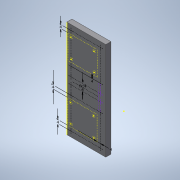
# Autodesk Inventor part: Z connection plate
Saved by Autodesk Inventor 2020 (Build 240168000, 168)
## iProperties
Created: 2019-05-25
Part Number: Z connection plate
Material: Generic
Document SubType Name: Modeling
Designer: LillaHunden
Density: 1 g/cm^3
Appearance: Default
Author: LillaHunden
Autodesk Inventor part; units mm, degrees
ref_plane "YZ Plane" through (0, 0, 0) normal (1, 0, 0) x (0, 1, 0)
ref_plane "XZ Plane" through (0, 0, 0) normal (0, 1, 0) x (-1, 0, 0)
ref_plane "XY Plane" through (0, 0, 0) normal (0, 0, 1) x (1, 0, 0)
sketch "Sketch1" plane through (0, 0, 0) normal (0, 0, 1) x (1, 0, 0)
  line L0 (-36.5524, -46.7459) -> (-66.2609, -46.7459) construction
  line L1 (-66.2609, -46.7459) -> (-66.2609, -56.6459) construction
  line L2 (-66.2609, -56.6459) -> (-1.9697, -56.6459) construction
  arc A0 (-1.9697, -56.6459) -> (0.0303, -54.6459) centre (-1.9697, -54.6459) ccw construction
  line L3 (0.0303, -54.6459) -> (0.0303, -27.2432) construction
  arc A1 (2.0303, -25.2432) -> (0.0303, -27.2432) centre (2.0303, -27.2432) ccw construction
  line L4 (2.0303, -25.2432) -> (9.9038, -25.2432) construction
  arc A2 (9.9038, -25.2432) -> (11.9038, -23.2432) centre (9.9038, -23.2432) ccw construction
  line L5 (11.9038, -23.2432) -> (11.9038, -14.7192) construction
  arc A3 (11.9038, -14.7192) -> (9.9038, -12.7192) centre (9.9038, -14.7192) ccw construction
  line L6 (9.9038, -12.7192) -> (2.0303, -12.7192) construction
  arc A4 (0.0303, -10.7192) -> (2.0303, -12.7192) centre (2.0303, -10.7192) ccw construction
  line L7 (0.0303, -10.7192) -> (0.0303, 56.6459) construction
  line L8 (-66.2609, -18.5459) -> (-36.5524, -18.5459) construction
  arc A5 (-30.8955, -24.2027) -> (-36.5524, -18.5459) centre (-33.7239, -21.3743) ccw construction
  line L9 (-30.8955, -24.2027) -> (-30.8955, -41.089) construction
  arc A6 (-36.5524, -46.7459) -> (-30.8955, -41.089) centre (-33.7239, -43.9175) ccw construction
  line L10 (-66.2609, 56.6459) -> (-20.9295, 56.6459)
  line L11 (-20.9295, 56.6459) -> (-20.9295, -56.6459)
  line L12 (-20.9295, -56.6459) -> (-66.2609, -56.6459)
  line L13 (-66.2609, -56.6459) -> (-66.2609, 56.6459)
  circle A7 centre (-26.9955, -4) radius 1.2295 projected
  circle A8 centre (-61.3755, 4) radius 1.2295 projected
  circle A9 centre (-26.9955, -50.6459) radius 1.2295 projected
  circle A10 centre (-61.3755, -14.6459) radius 1.2295 projected
  circle A11 centre (-26.9955, 14.6459) radius 1.2295 projected
  circle A12 centre (-26.9955, 50.6459) radius 1.2295 projected
  circle A13 centre (-61.3755, 50.6459) radius 1.2295 projected
  circle A14 centre (-61.3755, 14.6459) radius 1.2295 projected
  circle A15 centre (-26.9955, -14.6459) radius 1.2295 projected
  circle A16 centre (-61.3755, -50.6459) radius 1.2295 projected
  circle A17 centre (-26.9955, 4) radius 1.2295 projected
  circle A18 centre (-61.3755, -4) radius 1.2295 projected
  line L14 (-66.2609, 56.6459) -> (-66.2609, -18.5459) projected
  arc A19 (-30.8455, 41.089) -> (-36.5024, 46.7459) centre (-33.6739, 43.9175) ccw projected
  line L15 (-64.9755, 18.5459) -> (-64.9755, 46.7459) projected
  line L16 (-64.9755, 46.7459) -> (-36.5024, 46.7459) projected
  line L17 (0.0303, 56.6459) -> (-66.2609, 56.6459) projected
  line L18 (-30.8455, 41.089) -> (-30.8455, 24.252) projected
  arc A20 (-36.4527, 18.5459) -> (-30.8455, 24.252) centre (-33.6491, 21.3989) ccw projected
  line L19 (-36.4527, 18.5459) -> (-64.9755, 18.5459) projected
  point P0 (0, 0)
  point P1 (-64.9755, 18.5953)
  point P2 (-66.2609, 18.5953)
  constraints: 8 end point, 2 parallel, 1 horizontal, 1 perpendicular, 1 point on line
extrude "Extrusion1" add sketch "Sketch1" along normal blind 6 contours L10 L11 L12 L13 | A7 | A8 | A9 | A10 | A11 | A12 | A13 | A14 | A15 | A16 | A17 | A18 | L18 A20 L19 L15 L16 A19
sketch "Sketch2" plane through (0, 0, 6) normal (0, 0, 1) x (1, 0, 0)
  circle A0 centre (-34.2455, 22.0059) radius 1.621 construction
  circle A1 centre (-61.3755, 43.9159) radius 1.621 construction
  circle A2 centre (-60.8955, 22.0259) radius 1.621 construction
  circle A3 centre (-34.4255, 43.2959) radius 1.621 construction
  line L0 (-30.9455, 18.6459) -> (-64.8755, 18.6459) construction
  line L1 (-30.9455, 46.6459) -> (-30.9455, 18.6459) construction
  line L2 (-64.8755, 46.6459) -> (-30.9455, 46.6459) construction
  line L3 (-64.8755, 18.6459) -> (-64.8755, 46.6459) construction
  circle A4 centre (-61.6255, -22.0059) radius 1.621 construction
  circle A5 centre (-34.4955, -43.9159) radius 1.621 construction
  circle A6 centre (-34.9755, -22.0259) radius 1.621 construction
  circle A7 centre (-61.4455, -43.2959) radius 1.621 construction
  line L4 (-64.9255, -18.6459) -> (-30.9955, -18.6459) construction
  line L5 (-64.9255, -46.6459) -> (-64.9255, -18.6459) construction
  line L6 (-30.9955, -46.6459) -> (-64.9255, -46.6459) construction
  line L7 (-30.9955, -18.6459) -> (-30.9955, -46.6459) construction
  line L8 (-61.3755, 50.6459) -> (-26.9955, 50.6459) construction
  line L9 (-26.9955, 50.6459) -> (-26.9955, 14.6459) construction
  line L10 (-26.9955, 14.6459) -> (-61.3755, 14.6459) construction
  line L11 (-61.3755, 14.6459) -> (-61.3755, 50.6459) construction
  line L12 (-61.3755, -14.6459) -> (-26.9955, -14.6459) construction
  line L13 (-26.9955, -14.6459) -> (-26.9955, -50.6459) construction
  line L14 (-26.9955, -50.6459) -> (-61.3755, -50.6459) construction
  line L15 (-61.3755, -50.6459) -> (-61.3755, -14.6459) construction
  line L16 (-61.3755, 14.6459) -> (-26.9955, 14.6459) construction
  line L17 (-26.9955, 14.6459) -> (-26.9955, 4) construction
  line L18 (-26.9955, 4) -> (-61.3755, 4) construction
  line L19 (-61.3755, 4) -> (-61.3755, 14.6459) construction
  line L20 (-61.3755, -14.6459) -> (-26.9955, -14.6459) construction
  line L21 (-26.9955, -14.6459) -> (-26.9955, -4) construction
  line L22 (-26.9955, -4) -> (-61.3755, -4) construction
  line L23 (-61.3755, -4) -> (-61.3755, -14.6459) construction
  line L24 (-29.2136, 14.6459) -> (-29.2136, -14.6459) construction
  line L25 (-29.2136, 0) -> (-59.8245, 0) construction
  line L26 (-66.2609, 56.6459) -> (-66.2609, -56.6459) projected
  point P0 (0, 0)
  dimension "d2" = 4
  dimension "d3" = 4
  dimension "d4" = 4
  dimension "d5" = 4
  dimension "d6" = 4
  dimension "d7" = 4
  dimension "d8" = 4
  constraints: 36 end point, 12 coincident, 8 parallel, 5 horizontal, 5 perpendicular, 4 point on line, 1 midpoint, 1 vertical alignment
  measures "d2" distance between parallel lines of L4 L12
  measures "d3" distance between parallel lines of L14 L6
  measures "d4" distance between parallel lines of L7 L13
  measures "d5" distance between parallel lines of L10 L0
  measures "d6" distance between parallel lines of L2 L8
  measures "d7" distance between parallel lines of L25 L22
  measures "d8" distance between parallel lines of L25 L18
sketch "Sketch3" plane through (0, 0, 6) normal (0, 0, 1) x (1, 0, 0)
  point P0 (-26.9955, 50.6459)
  point P1 (-61.3755, 50.6459)
  point P2 (-26.9955, 14.6459)
  point P3 (-61.3755, 14.6459)
  point P4 (-61.3755, -14.6459)
  point P5 (-26.9955, -14.6459)
  point P6 (-26.9955, -50.6459)
  point P7 (-61.3755, -50.6459)
  point P8 (-61.3755, 4)
  point P9 (-26.9955, 4)
  point P10 (-26.9955, -4)
  point P11 (-61.3755, -4)
hole "Hole1" at (-26.9955, 50.6459, 6) at (-61.3755, 50.6459, 6) at (-26.9955, 14.6459, 6) at (-61.3755, 14.6459, 6) at (-61.3755, -14.6459, 6) at (-26.9955, -14.6459, 6) at (-26.9955, -50.6459, 6) at (-61.3755, -50.6459, 6) at (-61.3755, 4, 6) at (-26.9955, 4, 6) at (-26.9955, -4, 6) at (-61.3755, -4, 6) direction (0, 0, -1) diameter 3.6 depth 6 counterbore diameter 6.5 counterbore depth 3.4
sketch "Sketch4" plane through (0, 0, 6) normal (0, 0, 1) x (1, 0, 0)
  point P0 (-34.4255, 43.2959)
  point P1 (-61.3755, 43.9159)
  point P2 (-60.8955, 22.0259)
  point P3 (-34.2455, 22.0059)
hole "Hole3" at (-34.4255, 43.2959, 6) at (-61.3755, 43.9159, 6) at (-60.8955, 22.0259, 6) at (-34.2455, 22.0059, 6) direction (0, 0, -1) diameter 4.8 depth 6 counterbore diameter 8 counterbore depth 4.5
sketch "Sketch5" plane through (0, 0, 6) normal (0, 0, 1) x (1, 0, 0)
  point P0 (-61.6255, -22.0059)
  point P1 (-34.4955, -43.9159)
  point P2 (-34.9755, -22.0259)
  point P3 (-61.4455, -43.2959)
hole "Hole5" at (-61.6255, -22.0059, 6) at (-34.4955, -43.9159, 6) at (-34.9755, -22.0259, 6) at (-61.4455, -43.2959, 6) direction (0, 0, -1) diameter 4.8 depth 6 counterbore diameter 8 counterbore depth 4.5
equation "\"d8\" = d7"
body "Solid1"
